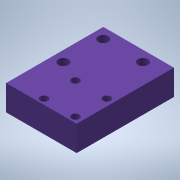
# Autodesk Inventor part: baseplate for combined beam steering mirror
Saved by Autodesk Inventor 2022 (Build 260153000, 153)
## iProperties
Created: 2013-10-22
Part Number: baseplate for combined beam steering mirror
Document SubType Name: Modeling
Designer: betzige
Density: 1 g/cm^3
Material: Generic
Appearance: Violet
Author: betzige
Autodesk Inventor part; units mm, degrees
ref_plane "YZ Plane" through (0, 0, 0) normal (1, 0, 0) x (0, 1, 0)
ref_plane "XZ Plane" through (0, 0, 0) normal (0, 1, 0) x (-1, 0, 0)
ref_plane "XY Plane" through (0, 0, 0) normal (0, 0, 1) x (1, 0, 0)
sketch "Sketch1" plane through (0, 0, 0) normal (0, 0, 1) x (1, 0, 0)
  line L0 (-22.5, 31) -> (22.5, 31)
  line L1 (22.5, 31) -> (22.5, -31)
  line L2 (22.5, -31) -> (-22.5, -31)
  line L3 (-22.5, -31) -> (-22.5, 31)
  point P0 (0, 0)
  dimension "d0" = 45
  dimension "d1" = 62
  dimension "d2" = 31
  dimension "d3" = 22.5
  constraints: 8 end point, 2 parallel, 1 horizontal, 1 perpendicular
  measures "d0" distance of L0.start L0.end
  measures "d1" distance of L2.end L0.start
  measures "d2" distance from line of point (0, 0) L0
  measures "d3" distance from line of point (0, 0) L3
extrude "Extrusion1" add sketch "Sketch1" along normal blind 16.2198
sketch "Sketch2" plane through (0, 0, 0) normal (0, 0, -1) x (-1, 0, 0)
  arc A0 (79.5379, 557.794) -> (67.0425, 570.2987) centre (67.0379, 557.7987) ccw projected
  line L0 (67.0425, 570.2987) -> (-365.1574, 570.4588) projected
  arc A1 (-365.1574, 570.4588) -> (-377.6621, 557.9635) centre (-365.1621, 557.9588) ccw projected
  line L1 (-377.6621, 557.9635) -> (-377.8787, -26.6365) projected
  arc A2 (-377.8787, -26.6365) -> (-365.3834, -39.1411) centre (-365.3787, -26.6411) ccw projected
  line L2 (-365.3834, -39.1411) -> (66.8166, -39.3013) projected
  arc A3 (66.8166, -39.3013) -> (79.3212, -26.8059) centre (66.8212, -26.8013) ccw projected
  line L3 (79.3212, -26.8059) -> (79.5379, 557.794) projected
  circle A4 centre (-339.5621, 557.7494) radius 2.5527 projected
  circle A5 centre (-314.1622, 557.7399) radius 2.5527 projected
  circle A6 centre (-288.7622, 557.7305) radius 2.5527 projected
  circle A7 centre (-263.3622, 557.7211) radius 2.5527 projected
  circle A8 centre (-237.9622, 557.7117) radius 2.5527 projected
  circle A9 centre (-212.5622, 557.7023) radius 2.5527 projected
  circle A10 centre (-187.1622, 557.6929) radius 2.5527 projected
  circle A11 centre (-161.7622, 557.6835) radius 2.5527 projected
  circle A12 centre (-136.3622, 557.674) radius 2.5527 projected
  circle A13 centre (-110.9622, 557.6646) radius 2.5527 projected
  circle A14 centre (-85.5622, 557.6552) radius 2.5527 projected
  circle A15 centre (-60.1622, 557.6458) radius 2.5527 projected
  circle A16 centre (-34.7622, 557.6364) radius 2.5527 projected
  circle A17 centre (-9.3622, 557.627) radius 2.5527 projected
  circle A18 centre (16.0378, 557.6176) radius 2.5527 projected
  circle A19 centre (41.4378, 557.6081) radius 2.5527 projected
  circle A20 centre (66.8378, 557.5987) radius 2.5527 projected
  circle A21 centre (-364.9716, 532.3588) radius 2.5527 projected
  circle A22 centre (-339.5716, 532.3494) radius 2.5527 projected
  circle A23 centre (-314.1716, 532.3399) radius 2.5527 projected
  circle A24 centre (-288.7716, 532.3305) radius 2.5527 projected
  circle A25 centre (-263.3716, 532.3211) radius 2.5527 projected
  circle A26 centre (-237.9716, 532.3117) radius 2.5527 projected
  circle A27 centre (-212.5716, 532.3023) radius 2.5527 projected
  circle A28 centre (-187.1716, 532.2929) radius 2.5527 projected
  circle A29 centre (-161.7716, 532.2835) radius 2.5527 projected
  circle A30 centre (-136.3716, 532.274) radius 2.5527 projected
  circle A31 centre (-110.9716, 532.2646) radius 2.5527 projected
  circle A32 centre (-85.5716, 532.2552) radius 2.5527 projected
  circle A33 centre (-60.1716, 532.2458) radius 2.5527 projected
  circle A34 centre (-34.7716, 532.2364) radius 2.5527 projected
  circle A35 centre (-9.3716, 532.227) radius 2.5527 projected
  circle A36 centre (16.0284, 532.2176) radius 2.5527 projected
  circle A37 centre (41.4284, 532.2081) radius 2.5527 projected
  circle A38 centre (66.8284, 532.1987) radius 2.5527 projected
  circle A39 centre (-364.981, 506.9588) radius 2.5527 projected
  circle A40 centre (-339.581, 506.9494) radius 2.5527 projected
  circle A41 centre (-314.181, 506.9399) radius 2.5527 projected
  circle A42 centre (-288.781, 506.9305) radius 2.5527 projected
  circle A43 centre (-263.381, 506.9211) radius 2.5527 projected
  circle A44 centre (-237.981, 506.9117) radius 2.5527 projected
  circle A45 centre (-212.581, 506.9023) radius 2.5527 projected
  circle A46 centre (-187.181, 506.8929) radius 2.5527 projected
  circle A47 centre (-161.781, 506.8835) radius 2.5527 projected
  circle A48 centre (-136.381, 506.874) radius 2.5527 projected
  circle A49 centre (-110.981, 506.8646) radius 2.5527 projected
  circle A50 centre (-85.581, 506.8552) radius 2.5527 projected
  circle A51 centre (-60.181, 506.8458) radius 2.5527 projected
  circle A52 centre (-34.781, 506.8364) radius 2.5527 projected
  circle A53 centre (-9.381, 506.827) radius 2.5527 projected
  circle A54 centre (16.019, 506.8176) radius 2.5527 projected
  circle A55 centre (41.419, 506.8082) radius 2.5527 projected
  circle A56 centre (66.819, 506.7987) radius 2.5527 projected
  circle A57 centre (-364.9904, 481.5588) radius 2.5527 projected
  circle A58 centre (-339.5904, 481.5494) radius 2.5527 projected
  circle A59 centre (-314.1904, 481.5399) radius 2.5527 projected
  circle A60 centre (-288.7904, 481.5305) radius 2.5527 projected
  circle A61 centre (-263.3904, 481.5211) radius 2.5527 projected
  circle A62 centre (-237.9904, 481.5117) radius 2.5527 projected
  circle A63 centre (-212.5904, 481.5023) radius 2.5527 projected
  circle A64 centre (-187.1904, 481.4929) radius 2.5527 projected
  circle A65 centre (-161.7904, 481.4835) radius 2.5527 projected
  circle A66 centre (-136.3904, 481.474) radius 2.5527 projected
  circle A67 centre (-110.9904, 481.4646) radius 2.5527 projected
  circle A68 centre (-85.5904, 481.4552) radius 2.5527 projected
  circle A69 centre (-60.1904, 481.4458) radius 2.5527 projected
  circle A70 centre (-34.7904, 481.4364) radius 2.5527 projected
  circle A71 centre (-9.3904, 481.427) radius 2.5527 projected
  circle A72 centre (16.0096, 481.4176) radius 2.5527 projected
  circle A73 centre (41.4096, 481.4082) radius 2.5527 projected
  circle A74 centre (66.8096, 481.3987) radius 2.5527 projected
  circle A75 centre (-364.9998, 456.1588) radius 2.5527 projected
  circle A76 centre (-339.5998, 456.1494) radius 2.5527 projected
  circle A77 centre (-314.1998, 456.1399) radius 2.5527 projected
  circle A78 centre (-288.7998, 456.1305) radius 2.5527 projected
  circle A79 centre (-263.3998, 456.1211) radius 2.5527 projected
  circle A80 centre (-237.9998, 456.1117) radius 2.5527 projected
  circle A81 centre (-212.5998, 456.1023) radius 2.5527 projected
  circle A82 centre (-187.1998, 456.0929) radius 2.5527 projected
  circle A83 centre (-161.7998, 456.0835) radius 2.5527 projected
  circle A84 centre (-136.3998, 456.074) radius 2.5527 projected
  circle A85 centre (-110.9998, 456.0646) radius 2.5527 projected
  circle A86 centre (-85.5998, 456.0552) radius 2.5527 projected
  circle A87 centre (-60.1998, 456.0458) radius 2.5527 projected
  circle A88 centre (-34.7998, 456.0364) radius 2.5527 projected
  circle A89 centre (-9.3998, 456.027) radius 2.5527 projected
  circle A90 centre (16.0002, 456.0176) radius 2.5527 projected
  circle A91 centre (41.4002, 456.0082) radius 2.5527 projected
  circle A92 centre (66.8002, 455.9987) radius 2.5527 projected
  circle A93 centre (-365.0092, 430.7588) radius 2.5527 projected
  circle A94 centre (-339.6092, 430.7494) radius 2.5527 projected
  circle A95 centre (-314.2092, 430.7399) radius 2.5527 projected
  circle A96 centre (-288.8092, 430.7305) radius 2.5527 projected
  circle A97 centre (-263.4092, 430.7211) radius 2.5527 projected
  circle A98 centre (-238.0092, 430.7117) radius 2.5527 projected
  circle A99 centre (-212.6092, 430.7023) radius 2.5527 projected
  circle A100 centre (-187.2092, 430.6929) radius 2.5527 projected
  circle A101 centre (-161.8092, 430.6835) radius 2.5527 projected
  circle A102 centre (-136.4092, 430.6741) radius 2.5527 projected
  circle A103 centre (-111.0092, 430.6646) radius 2.5527 projected
  circle A104 centre (-85.6092, 430.6552) radius 2.5527 projected
  circle A105 centre (-60.2092, 430.6458) radius 2.5527 projected
  circle A106 centre (-34.8092, 430.6364) radius 2.5527 projected
  circle A107 centre (-9.4092, 430.627) radius 2.5527 projected
  circle A108 centre (15.9908, 430.6176) radius 2.5527 projected
  circle A109 centre (41.3908, 430.6082) radius 2.5527 projected
  circle A110 centre (66.7908, 430.5987) radius 2.5527 projected
  circle A111 centre (-365.0186, 405.3588) radius 2.5527 projected
  circle A112 centre (-339.6186, 405.3494) radius 2.5527 projected
  circle A113 centre (-314.2186, 405.3399) radius 2.5527 projected
  circle A114 centre (-288.8186, 405.3305) radius 2.5527 projected
  circle A115 centre (-263.4186, 405.3211) radius 2.5527 projected
  circle A116 centre (-238.0186, 405.3117) radius 2.5527 projected
  circle A117 centre (-212.6186, 405.3023) radius 2.5527 projected
  circle A118 centre (-187.2186, 405.2929) radius 2.5527 projected
  circle A119 centre (-161.8186, 405.2835) radius 2.5527 projected
  circle A120 centre (-136.4186, 405.2741) radius 2.5527 projected
  circle A121 centre (-111.0186, 405.2646) radius 2.5527 projected
  circle A122 centre (-85.6186, 405.2552) radius 2.5527 projected
  circle A123 centre (-60.2186, 405.2458) radius 2.5527 projected
  circle A124 centre (-34.8187, 405.2364) radius 2.5527 projected
  circle A125 centre (-9.4187, 405.227) radius 2.5527 projected
  circle A126 centre (15.9813, 405.2176) radius 2.5527 projected
  circle A127 centre (41.3813, 405.2082) radius 2.5527 projected
  circle A128 centre (66.7813, 405.1987) radius 2.5527 projected
  circle A129 centre (-365.028, 379.9588) radius 2.5527 projected
  circle A130 centre (-339.628, 379.9494) radius 2.5527 projected
  circle A131 centre (-314.228, 379.94) radius 2.5527 projected
  circle A132 centre (-288.828, 379.9305) radius 2.5527 projected
  circle A133 centre (-263.428, 379.9211) radius 2.5527 projected
  circle A134 centre (-238.0281, 379.9117) radius 2.5527 projected
  circle A135 centre (-212.6281, 379.9023) radius 2.5527 projected
  circle A136 centre (-187.2281, 379.8929) radius 2.5527 projected
  circle A137 centre (-161.8281, 379.8835) radius 2.5527 projected
  circle A138 centre (-136.4281, 379.8741) radius 2.5527 projected
  circle A139 centre (-111.0281, 379.8646) radius 2.5527 projected
  circle A140 centre (-85.6281, 379.8552) radius 2.5527 projected
  circle A141 centre (-60.2281, 379.8458) radius 2.5527 projected
  circle A142 centre (-34.8281, 379.8364) radius 2.5527 projected
  circle A143 centre (-9.4281, 379.827) radius 2.5527 projected
  circle A144 centre (15.9719, 379.8176) radius 2.5527 projected
  circle A145 centre (41.3719, 379.8082) radius 2.5527 projected
  circle A146 centre (66.7719, 379.7987) radius 2.5527 projected
  circle A147 centre (-365.0375, 354.5588) radius 2.5527 projected
  circle A148 centre (-339.6375, 354.5494) radius 2.5527 projected
  circle A149 centre (-314.2375, 354.54) radius 2.5527 projected
  circle A150 centre (-288.8375, 354.5305) radius 2.5527 projected
  circle A151 centre (-263.4375, 354.5211) radius 2.5527 projected
  circle A152 centre (-238.0375, 354.5117) radius 2.5527 projected
  circle A153 centre (-212.6375, 354.5023) radius 2.5527 projected
  circle A154 centre (-187.2375, 354.4929) radius 2.5527 projected
  circle A155 centre (-161.8375, 354.4835) radius 2.5527 projected
  circle A156 centre (-136.4375, 354.4741) radius 2.5527 projected
  circle A157 centre (-111.0375, 354.4646) radius 2.5527 projected
  circle A158 centre (-85.6375, 354.4552) radius 2.5527 projected
  circle A159 centre (-60.2375, 354.4458) radius 2.5527 projected
  circle A160 centre (-34.8375, 354.4364) radius 2.5527 projected
  circle A161 centre (-9.4375, 354.427) radius 2.5527 projected
  circle A162 centre (15.9625, 354.4176) radius 2.5527 projected
  circle A163 centre (41.3625, 354.4082) radius 2.5527 projected
  circle A164 centre (66.7625, 354.3987) radius 2.5527 projected
  circle A165 centre (-365.0469, 329.1588) radius 2.5527 projected
  circle A166 centre (-339.6469, 329.1494) radius 2.5527 projected
  circle A167 centre (-314.2469, 329.14) radius 2.5527 projected
  circle A168 centre (-288.8469, 329.1305) radius 2.5527 projected
  circle A169 centre (-263.4469, 329.1211) radius 2.5527 projected
  circle A170 centre (-238.0469, 329.1117) radius 2.5527 projected
  circle A171 centre (-212.6469, 329.1023) radius 2.5527 projected
  circle A172 centre (-187.2469, 329.0929) radius 2.5527 projected
  circle A173 centre (-161.8469, 329.0835) radius 2.5527 projected
  circle A174 centre (-136.4469, 329.0741) radius 2.5527 projected
  circle A175 centre (-111.0469, 329.0646) radius 2.5527 projected
  circle A176 centre (-85.6469, 329.0552) radius 2.5527 projected
  circle A177 centre (-60.2469, 329.0458) radius 2.5527 projected
  circle A178 centre (-34.8469, 329.0364) radius 2.5527 projected
  circle A179 centre (-9.4469, 329.027) radius 2.5527 projected
  circle A180 centre (15.9531, 329.0176) radius 2.5527 projected
  circle A181 centre (41.3531, 329.0082) radius 2.5527 projected
  circle A182 centre (66.7531, 328.9987) radius 2.5527 projected
  circle A183 centre (-365.0563, 303.7588) radius 2.5527 projected
  circle A184 centre (-339.6563, 303.7494) radius 2.5527 projected
  circle A185 centre (-314.2563, 303.74) radius 2.5527 projected
  circle A186 centre (-288.8563, 303.7305) radius 2.5527 projected
  circle A187 centre (-263.4563, 303.7211) radius 2.5527 projected
  circle A188 centre (-238.0563, 303.7117) radius 2.5527 projected
  circle A189 centre (-212.6563, 303.7023) radius 2.5527 projected
  circle A190 centre (-187.2563, 303.6929) radius 2.5527 projected
  circle A191 centre (-161.8563, 303.6835) radius 2.5527 projected
  circle A192 centre (-136.4563, 303.6741) radius 2.5527 projected
  circle A193 centre (-111.0563, 303.6646) radius 2.5527 projected
  circle A194 centre (-85.6563, 303.6552) radius 2.5527 projected
  circle A195 centre (-60.2563, 303.6458) radius 2.5527 projected
  circle A196 centre (-34.8563, 303.6364) radius 2.5527 projected
  circle A197 centre (-9.4563, 303.627) radius 2.5527 projected
  circle A198 centre (15.9437, 303.6176) radius 2.5527 projected
  circle A199 centre (41.3437, 303.6082) radius 2.5527 projected
  circle A200 centre (66.7437, 303.5988) radius 2.5527 projected
  circle A201 centre (-365.0657, 278.3588) radius 2.5527 projected
  circle A202 centre (-339.6657, 278.3494) radius 2.5527 projected
  circle A203 centre (-314.2657, 278.34) radius 2.5527 projected
  circle A204 centre (-288.8657, 278.3305) radius 2.5527 projected
  circle A205 centre (-263.4657, 278.3211) radius 2.5527 projected
  circle A206 centre (-238.0657, 278.3117) radius 2.5527 projected
  circle A207 centre (-212.6657, 278.3023) radius 2.5527 projected
  circle A208 centre (-187.2657, 278.2929) radius 2.5527 projected
  circle A209 centre (-161.8657, 278.2835) radius 2.5527 projected
  circle A210 centre (-136.4657, 278.2741) radius 2.5527 projected
  circle A211 centre (-111.0657, 278.2646) radius 2.5527 projected
  circle A212 centre (-85.6657, 278.2552) radius 2.5527 projected
  circle A213 centre (-60.2657, 278.2458) radius 2.5527 projected
  circle A214 centre (-34.8657, 278.2364) radius 2.5527 projected
  circle A215 centre (-9.4657, 278.227) radius 2.5527 projected
  circle A216 centre (15.9343, 278.2176) radius 2.5527 projected
  circle A217 centre (41.3343, 278.2082) radius 2.5527 projected
  circle A218 centre (66.7343, 278.1988) radius 2.5527 projected
  circle A219 centre (-365.0751, 252.9588) radius 2.5527 projected
  circle A220 centre (-339.6751, 252.9494) radius 2.5527 projected
  circle A221 centre (-314.2751, 252.94) radius 2.5527 projected
  circle A222 centre (-288.8751, 252.9305) radius 2.5527 projected
  circle A223 centre (-263.4751, 252.9211) radius 2.5527 projected
  circle A224 centre (-238.0751, 252.9117) radius 2.5527 projected
  circle A225 centre (-212.6751, 252.9023) radius 2.5527 projected
  circle A226 centre (-187.2751, 252.8929) radius 2.5527 projected
  circle A227 centre (-161.8751, 252.8835) radius 2.5527 projected
  circle A228 centre (-136.4751, 252.8741) radius 2.5527 projected
  circle A229 centre (-111.0751, 252.8647) radius 2.5527 projected
  circle A230 centre (-85.6751, 252.8552) radius 2.5527 projected
  circle A231 centre (-60.2751, 252.8458) radius 2.5527 projected
  circle A232 centre (-34.8751, 252.8364) radius 2.5527 projected
  circle A233 centre (-9.4751, 252.827) radius 2.5527 projected
  circle A234 centre (15.9249, 252.8176) radius 2.5527 projected
  circle A235 centre (41.3249, 252.8082) radius 2.5527 projected
  circle A236 centre (66.7249, 252.7988) radius 2.5527 projected
  circle A237 centre (-365.0845, 227.5588) radius 2.5527 projected
  circle A238 centre (-339.6845, 227.5494) radius 2.5527 projected
  circle A239 centre (-314.2845, 227.54) radius 2.5527 projected
  circle A240 centre (-288.8845, 227.5305) radius 2.5527 projected
  circle A241 centre (-263.4845, 227.5211) radius 2.5527 projected
  circle A242 centre (-238.0845, 227.5117) radius 2.5527 projected
  circle A243 centre (-212.6845, 227.5023) radius 2.5527 projected
  circle A244 centre (-187.2845, 227.4929) radius 2.5527 projected
  circle A245 centre (-161.8845, 227.4835) radius 2.5527 projected
  circle A246 centre (-136.4845, 227.4741) radius 2.5527 projected
  circle A247 centre (-111.0845, 227.4647) radius 2.5527 projected
  circle A248 centre (-85.6845, 227.4552) radius 2.5527 projected
  circle A249 centre (-60.2845, 227.4458) radius 2.5527 projected
  circle A250 centre (-34.8845, 227.4364) radius 2.5527 projected
  circle A251 centre (-9.4845, 227.427) radius 2.5527 projected
  circle A252 centre (15.9154, 227.4176) radius 2.5527 projected
  circle A253 centre (41.3154, 227.4082) radius 2.5527 projected
  circle A254 centre (66.7154, 227.3988) radius 2.5527 projected
  circle A255 centre (-365.0939, 202.1588) radius 2.5527 projected
  circle A256 centre (-339.6939, 202.1494) radius 2.5527 projected
  circle A257 centre (-314.2939, 202.14) radius 2.5527 projected
  circle A258 centre (-288.8939, 202.1305) radius 2.5527 projected
  circle A259 centre (-263.4939, 202.1211) radius 2.5527 projected
  circle A260 centre (-238.0939, 202.1117) radius 2.5527 projected
  circle A261 centre (-212.6939, 202.1023) radius 2.5527 projected
  circle A262 centre (-187.294, 202.0929) radius 2.5527 projected
  circle A263 centre (-161.894, 202.0835) radius 2.5527 projected
  circle A264 centre (-136.494, 202.0741) radius 2.5527 projected
  circle A265 centre (-111.094, 202.0647) radius 2.5527 projected
  circle A266 centre (-85.694, 202.0552) radius 2.5527 projected
  circle A267 centre (-60.294, 202.0458) radius 2.5527 projected
  circle A268 centre (-34.894, 202.0364) radius 2.5527 projected
  circle A269 centre (-9.494, 202.027) radius 2.5527 projected
  circle A270 centre (15.906, 202.0176) radius 2.5527 projected
  circle A271 centre (41.306, 202.0082) radius 2.5527 projected
  circle A272 centre (66.706, 201.9988) radius 2.5527 projected
  circle A273 centre (-365.1034, 176.7588) radius 2.5527 projected
  circle A274 centre (-339.7034, 176.7494) radius 2.5527 projected
  circle A275 centre (-314.3034, 176.74) radius 2.5527 projected
  circle A276 centre (-288.9034, 176.7306) radius 2.5527 projected
  circle A277 centre (-263.5034, 176.7211) radius 2.5527 projected
  circle A278 centre (-238.1034, 176.7117) radius 2.5527 projected
  circle A279 centre (-212.7034, 176.7023) radius 2.5527 projected
  circle A280 centre (-187.3034, 176.6929) radius 2.5527 projected
  circle A281 centre (-161.9034, 176.6835) radius 2.5527 projected
  circle A282 centre (-136.5034, 176.6741) radius 2.5527 projected
  circle A283 centre (-111.1034, 176.6647) radius 2.5527 projected
  circle A284 centre (-85.7034, 176.6552) radius 2.5527 projected
  circle A285 centre (-60.3034, 176.6458) radius 2.5527 projected
  circle A286 centre (-34.9034, 176.6364) radius 2.5527 projected
  circle A287 centre (-9.5034, 176.627) radius 2.5527 projected
  circle A288 centre (15.8966, 176.6176) radius 2.5527 projected
  circle A289 centre (41.2966, 176.6082) radius 2.5527 projected
  circle A290 centre (66.6966, 176.5988) radius 2.5527 projected
  circle A291 centre (-365.1128, 151.3588) radius 2.5527 projected
  circle A292 centre (-339.7128, 151.3494) radius 2.5527 projected
  circle A293 centre (-314.3128, 151.34) radius 2.5527 projected
  circle A294 centre (-288.9128, 151.3306) radius 2.5527 projected
  circle A295 centre (-263.5128, 151.3211) radius 2.5527 projected
  circle A296 centre (-238.1128, 151.3117) radius 2.5527 projected
  circle A297 centre (-212.7128, 151.3023) radius 2.5527 projected
  circle A298 centre (-187.3128, 151.2929) radius 2.5527 projected
  circle A299 centre (-161.9128, 151.2835) radius 2.5527 projected
  circle A300 centre (-136.5128, 151.2741) radius 2.5527 projected
  circle A301 centre (-111.1128, 151.2647) radius 2.5527 projected
  circle A302 centre (-85.7128, 151.2552) radius 2.5527 projected
  circle A303 centre (-60.3128, 151.2458) radius 2.5527 projected
  circle A304 centre (-34.9128, 151.2364) radius 2.5527 projected
  circle A305 centre (-9.5128, 151.227) radius 2.5527 projected
  circle A306 centre (15.8872, 151.2176) radius 2.5527 projected
  circle A307 centre (41.2872, 151.2082) radius 2.5527 projected
  circle A308 centre (66.6872, 151.1988) radius 2.5527 projected
  circle A309 centre (-365.1222, 125.9588) radius 2.5527 projected
  circle A310 centre (-339.7222, 125.9494) radius 2.5527 projected
  circle A311 centre (-314.3222, 125.94) radius 2.5527 projected
  circle A312 centre (-288.9222, 125.9306) radius 2.5527 projected
  circle A313 centre (-263.5222, 125.9211) radius 2.5527 projected
  circle A314 centre (-238.1222, 125.9117) radius 2.5527 projected
  circle A315 centre (-212.7222, 125.9023) radius 2.5527 projected
  circle A316 centre (-187.3222, 125.8929) radius 2.5527 projected
  circle A317 centre (-161.9222, 125.8835) radius 2.5527 projected
  circle A318 centre (-136.5222, 125.8741) radius 2.5527 projected
  circle A319 centre (-111.1222, 125.8647) radius 2.5527 projected
  circle A320 centre (-85.7222, 125.8552) radius 2.5527 projected
  circle A321 centre (-60.3222, 125.8458) radius 2.5527 projected
  circle A322 centre (-34.9222, 125.8364) radius 2.5527 projected
  circle A323 centre (-9.5222, 125.827) radius 2.5527 projected
  circle A324 centre (15.8778, 125.8176) radius 2.5527 projected
  circle A325 centre (41.2778, 125.8082) radius 2.5527 projected
  circle A326 centre (66.6778, 125.7988) radius 2.5527 projected
  circle A327 centre (-365.1316, 100.5588) radius 2.5527 projected
  circle A328 centre (-339.7316, 100.5494) radius 2.5527 projected
  circle A329 centre (-314.3316, 100.54) radius 2.5527 projected
  circle A330 centre (-288.9316, 100.5306) radius 2.5527 projected
  circle A331 centre (-263.5316, 100.5211) radius 2.5527 projected
  circle A332 centre (-238.1316, 100.5117) radius 2.5527 projected
  circle A333 centre (-212.7316, 100.5023) radius 2.5527 projected
  circle A334 centre (-187.3316, 100.4929) radius 2.5527 projected
  circle A335 centre (-161.9316, 100.4835) radius 2.5527 projected
  circle A336 centre (-136.5316, 100.4741) radius 2.5527 projected
  circle A337 centre (-111.1316, 100.4647) radius 2.5527 projected
  circle A338 centre (-85.7316, 100.4552) radius 2.5527 projected
  circle A339 centre (-60.3316, 100.4458) radius 2.5527 projected
  circle A340 centre (-34.9316, 100.4364) radius 2.5527 projected
  circle A341 centre (-9.5316, 100.427) radius 2.5527 projected
  circle A342 centre (15.8684, 100.4176) radius 2.5527 projected
  circle A343 centre (41.2684, 100.4082) radius 2.5527 projected
  circle A344 centre (66.6684, 100.3988) radius 2.5527 projected
  circle A345 centre (-365.141, 75.1588) radius 2.5527 projected
  circle A346 centre (-339.741, 75.1494) radius 2.5527 projected
  circle A347 centre (-314.341, 75.14) radius 2.5527 projected
  circle A348 centre (-288.941, 75.1306) radius 2.5527 projected
  circle A349 centre (-263.541, 75.1211) radius 2.5527 projected
  circle A350 centre (-238.141, 75.1117) radius 2.5527 projected
  circle A351 centre (-212.741, 75.1023) radius 2.5527 projected
  circle A352 centre (-187.341, 75.0929) radius 2.5527 projected
  circle A353 centre (-161.941, 75.0835) radius 2.5527 projected
  circle A354 centre (-136.541, 75.0741) radius 2.5527 projected
  circle A355 centre (-111.141, 75.0647) radius 2.5527 projected
  circle A356 centre (-85.741, 75.0552) radius 2.5527 projected
  circle A357 centre (-60.341, 75.0458) radius 2.5527 projected
  circle A358 centre (-34.941, 75.0364) radius 2.5527 projected
  circle A359 centre (-9.541, 75.027) radius 2.5527 projected
  circle A360 centre (15.859, 75.0176) radius 2.5527 projected
  circle A361 centre (41.259, 75.0082) radius 2.5527 projected
  circle A362 centre (66.659, 74.9988) radius 2.5527 projected
  circle A363 centre (-365.1504, 49.7588) radius 2.5527 projected
  circle A364 centre (-339.7504, 49.7494) radius 2.5527 projected
  circle A365 centre (-314.3504, 49.74) radius 2.5527 projected
  circle A366 centre (-288.9504, 49.7306) radius 2.5527 projected
  circle A367 centre (-263.5504, 49.7211) radius 2.5527 projected
  circle A368 centre (-238.1504, 49.7117) radius 2.5527 projected
  circle A369 centre (-212.7504, 49.7023) radius 2.5527 projected
  circle A370 centre (-187.3504, 49.6929) radius 2.5527 projected
  circle A371 centre (-161.9504, 49.6835) radius 2.5527 projected
  circle A372 centre (-136.5504, 49.6741) radius 2.5527 projected
  circle A373 centre (-111.1504, 49.6647) radius 2.5527 projected
  circle A374 centre (-85.7504, 49.6553) radius 2.5527 projected
  circle A375 centre (-60.3504, 49.6458) radius 2.5527 projected
  circle A376 centre (-34.9504, 49.6364) radius 2.5527 projected
  circle A377 centre (-9.5504, 49.627) radius 2.5527 projected
  circle A378 centre (15.8496, 49.6176) radius 2.5527 projected
  circle A379 centre (41.2496, 49.6082) radius 2.5527 projected
  circle A380 centre (66.6496, 49.5988) radius 2.5527 projected
  circle A381 centre (-365.1598, 24.3588) radius 2.5527 projected
  circle A382 centre (-339.7598, 24.3494) radius 2.5527 projected
  circle A383 centre (-314.3598, 24.34) radius 2.5527 projected
  circle A384 centre (-288.9598, 24.3306) radius 2.5527 projected
  circle A385 centre (-263.5598, 24.3211) radius 2.5527 projected
  circle A386 centre (-238.1598, 24.3117) radius 2.5527 projected
  circle A387 centre (-212.7598, 24.3023) radius 2.5527 projected
  circle A388 centre (-187.3598, 24.2929) radius 2.5527 projected
  circle A389 centre (-161.9598, 24.2835) radius 2.5527 projected
  circle A390 centre (-136.5598, 24.2741) radius 2.5527 projected
  circle A391 centre (-111.1599, 24.2647) radius 2.5527 projected
  circle A392 centre (-85.7599, 24.2553) radius 2.5527 projected
  circle A393 centre (-60.3599, 24.2458) radius 2.5527 projected
  circle A394 centre (-34.9599, 24.2364) radius 2.5527 projected
  circle A395 centre (-9.5599, 24.227) radius 2.5527 projected
  circle A396 centre (15.8401, 24.2176) radius 2.5527 projected
  circle A397 centre (41.2401, 24.2082) radius 2.5527 projected
  circle A398 centre (66.6401, 24.1988) radius 2.5527 projected
  circle A399 centre (-365.1692, -1.0412) radius 2.5527 projected
  circle A400 centre (-339.7692, -1.0506) radius 2.5527 projected
  circle A401 centre (-314.3693, -1.06) radius 2.5527 projected
  circle A402 centre (-288.9693, -1.0694) radius 2.5527 projected
  circle A403 centre (-263.5693, -1.0789) radius 2.5527 projected
  circle A404 centre (-238.1693, -1.0883) radius 2.5527 projected
  circle A405 centre (-212.7693, -1.0977) radius 2.5527 projected
  circle A406 centre (-187.3693, -1.1071) radius 2.5527 projected
  circle A407 centre (-161.9693, -1.1165) radius 2.5527 projected
  circle A408 centre (-136.5693, -1.1259) radius 2.5527 projected
  circle A409 centre (-111.1693, -1.1353) radius 2.5527 projected
  circle A410 centre (-85.7693, -1.1447) radius 2.5527 projected
  circle A411 centre (-60.3693, -1.1542) radius 2.5527 projected
  circle A412 centre (-34.9693, -1.1636) radius 2.5527 projected
  circle A413 centre (-9.5693, -1.173) radius 2.5527 projected
  circle A414 centre (15.8307, -1.1824) radius 2.5527 projected
  circle A415 centre (41.2307, -1.1918) radius 2.5527 projected
  circle A416 centre (66.6307, -1.2012) radius 2.5527 projected
  circle A417 centre (-365.1787, -26.4412) radius 2.5527 projected
  circle A418 centre (-339.7787, -26.4506) radius 2.5527 projected
  circle A419 centre (-314.3787, -26.46) radius 2.5527 projected
  circle A420 centre (-288.9787, -26.4694) radius 2.5527 projected
  circle A421 centre (-263.5787, -26.4788) radius 2.5527 projected
  circle A422 centre (-238.1787, -26.4883) radius 2.5527 projected
  circle A423 centre (-212.7787, -26.4977) radius 2.5527 projected
  circle A424 centre (-187.3787, -26.5071) radius 2.5527 projected
  circle A425 centre (-161.9787, -26.5165) radius 2.5527 projected
  circle A426 centre (-136.5787, -26.5259) radius 2.5527 projected
  circle A427 centre (-111.1787, -26.5353) radius 2.5527 projected
  circle A428 centre (-85.7787, -26.5447) radius 2.5527 projected
  circle A429 centre (-60.3787, -26.5542) radius 2.5527 projected
  circle A430 centre (-34.9787, -26.5636) radius 2.5527 projected
  circle A431 centre (-9.5787, -26.573) radius 2.5527 projected
  circle A432 centre (15.8213, -26.5824) radius 2.5527 projected
  circle A433 centre (41.2213, -26.5918) radius 2.5527 projected
  circle A434 centre (66.6213, -26.6012) radius 2.5527 projected
  circle A435 centre (-364.9621, 557.7588) radius 2.5527 projected
  point P0 (0, 0)
hole "Hole1" at (9.5599, 24.227, 0) at (-15.8401, 24.2176, 0) at (-15.8307, -1.1824, 0) direction (0, 0, 1) diameter 6.35 end through all counterbore diameter 9.652 counterbore depth 6.5
sketch "Sketch3" plane through (0, 0, 16.2198) normal (0, 0, 1) x (1, 0, 0)
  circle A0 centre (18.2032, -27.5) radius 0.889 projected
  circle A1 centre (-1.7968, -27.5) radius 1.0922 projected
  line L0 (20.7032, -5.508) -> (20.7032, -5) projected
  line L1 (20.7032, -5) -> (-4.2967, -5.0001) projected
  line L2 (-4.2967, -5.0001) -> (-4.2967, -30) projected
  line L3 (-4.2967, -30) -> (20.7032, -30) projected
  line L4 (20.7032, -30) -> (20.7032, -29.492) projected
  line L5 (20.7032, -29.492) -> (21.008, -29.492) projected
  line L6 (21.008, -5.508) -> (21.008, -29.492) projected
  line L7 (20.7032, -5.508) -> (21.008, -5.508) projected
  circle A2 centre (18.2032, -7.5) radius 0.889 projected
  circle A3 centre (-1.7968, -7.5) radius 0.889 projected
  circle A4 centre (18.2032, -27.5) radius 0.889 projected
  circle A5 centre (-1.7968, -27.5) radius 0.889 projected
  circle A6 centre (14.5532, -11.15) radius 1.7272 projected
  circle A7 centre (1.8532, -11.15) radius 1.7272 projected
  circle A8 centre (14.5532, -23.85) radius 1.7272 projected
  circle A9 centre (1.8532, -23.85) radius 1.7272 projected
  circle A10 centre (8.2032, -17.5) radius 1.7272 projected
  point P0 (0, 0)
hole "Hole2" at (18.2032, -7.5, 16.2198) at (-1.7968, -7.5, 16.2198) at (-1.7968, -27.5, 16.2198) at (18.2032, -27.5, 16.2198) direction (0, 0, -1) diameter 2.1844 end through all counterbore diameter 4.826 counterbore depth 11.28
body "Solid1"
